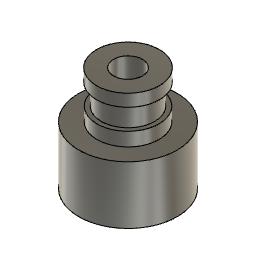
Stem_Adaptor (Autodesk Fusion 360 design; units mm, degrees)
Autodesk Fusion 360 part; units mm, degrees
sketch "Sketch1" plane through (0, 0, 0) normal (0, 1, 0) x (1, 0, 0)
  line L0 (0, 0) -> (0, -3.175)
  line L1 (0, -3.175) -> (0.9525, -3.175)
  line L2 (0, 0) -> (1.4922, 0)
  line L3 (0.9525, -3.175) -> (0.9525, -2.8051)
  line L4 (0.9525, -2.8051) -> (0.8097, -2.8051)
  line L5 (1.4922, 0) -> (1.4922, -1.7532)
  line L6 (0.8097, -2.8051) -> (0.8097, -2.1648)
  line L7 (0.8097, -2.1648) -> (0.94, -2.1648)
  line L8 (0.94, -2.1648) -> (0.94, -1.7532)
  line L9 (0.94, -1.7532) -> (1.4922, -1.7532)
  dimension "d1" = 3.175
  dimension "d3" = 1.4922
  constraint coincident L0.start L2.start
  constraint vertical L0
  constraint perpendicular L0 L1
  constraint perpendicular L0 L2
  constraint perpendicular L1 L3
  constraint perpendicular L3 L4
  constraint perpendicular L2 L5
  constraint perpendicular L4 L6
  constraint perpendicular L6 L7
  constraint perpendicular L7 L8
  constraint perpendicular L5 L9
  measures "d1" distance of L0.start L0.end
  measures "d3" distance of L0.start L2.end
revolve "Revolve1" add sketch "Sketch1" angle 360 about axis through (0, 0, 0) along (0, 0, 1)
sketch "Sketch2" plane through (0, 0, 3.175) normal (0, 0, 1) x (-1, 0, 0)
  circle A0 centre (0, 0) radius 0.9525
  circle A1 centre (0, 0) radius 0.4382
  dimension "d6" = 0.8763
  constraint coincident A0.centre A1.centre
  measures "d6" diameter of A1
extrude "Extrude1" cut sketch "Sketch2" against normal blind 2.54 contours A1
equation "d3 = ( 0.1175 / 2 ) * 1 in"
